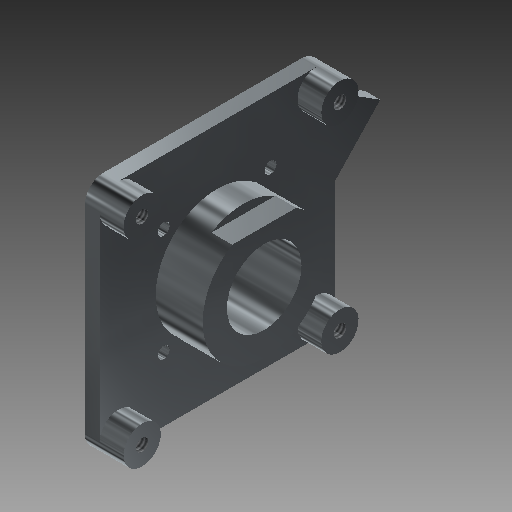
# Autodesk Inventor part: Face Plate
Saved by Autodesk Inventor 2017 (Build 210142000, 142)
## iProperties
Created: 2012-08-06
Part Number: Face Plate
Material: PC/ABS Plastic
Document SubType Name: Modeling
Designer: John
Density: 1.493 g/cm^3
Mass: 11.4166 g
Surface Area: 57.4511 cm^2
Volume: 7.64678 cm^3
Appearance: Zinc
Author: John
Autodesk Inventor part; units mm, degrees
ref_plane "YZ Plane" through (0, 0, 0) normal (1, 0, 0) x (0, 1, 0)
ref_plane "XZ Plane" through (0, 0, 0) normal (0, 1, 0) x (-1, 0, 0)
ref_plane "XY Plane" through (0, 0, 0) normal (0, 0, 1) x (1, 0, 0)
sketch "Sketch1" plane through (0, 0, 0) normal (1, 0, 0) x (0, 1, 0)
  line L0 (0, 0) -> (40.005, 0)
  line L1 (40.005, 0) -> (40.005, 40.005)
  line L2 (40.005, 40.005) -> (0, 40.005)
  line L3 (0, 40.005) -> (0, 0)
  dimension "d0" = 40.005
  dimension "d1" = 40.005
  constraints: 8 end point, 2 parallel, 1 horizontal, 1 perpendicular
  measures "d0" distance of L2.end L1.end
  measures "d1" distance of L0.end L1.end
extrude "Extrusion1" add sketch "Sketch1" along normal blind 2.54
fillet "Fillet1" radius 3.175 4 edges at (1.27, 40.005, 40.005) (1.27, 0, 40.005) (1.27, 0, 0) (1.27, 40.005, 0)
sketch "Sketch2" plane through (2.54, 0, 0) normal (1, 0, 0) x (0, 0, -1)
  arc A0 (0, 36.83) -> (-3.175, 40.005) centre (-3.175, 36.83) ccw projected
  arc A1 (-36.83, 40.005) -> (-40.005, 36.83) centre (-36.83, 36.83) ccw projected
  arc A2 (-40.005, 3.175) -> (-36.83, 0) centre (-36.83, 3.175) ccw projected
  arc A3 (-3.175, 0) -> (0, 3.175) centre (-3.175, 3.175) ccw projected
  circle A4 centre (-36.83, 3.175) radius 3.175
  circle A5 centre (-36.83, 36.83) radius 3.175
  circle A6 centre (-3.175, 36.83) radius 3.175
  circle A7 centre (-3.175, 3.175) radius 3.175
  point P0 (0, 0)
  constraints: 4 coincident, 3 horizontal alignment, 1 centre point, 1 concentric, 6 other
extrude "Extrusion2" add sketch "Sketch2" along normal blind 4.064
sketch "Sketch3" plane through (6.604, 3.175, 36.83) normal (1, 0, 0) x (0, 0, -1)
  circle A0 centre (0, 0) radius 3.175 projected
  circle A1 centre (0, 33.655) radius 3.175 projected
  circle A2 centre (33.655, 33.655) radius 3.175 projected
  circle A3 centre (33.655, 0) radius 3.175 projected
  point P0 (36.83, -3.175)
hole "Hole1" at (6.604, 36.83, 36.83) at (6.604, 36.83, 3.175) at (6.604, 3.175, 3.175) at (6.604, 3.175, 36.83) direction (-1, 0, 0) diameter 2.159 end through all
sketch "Sketch4" plane through (2.54, 0, 0) normal (1, 0, 0) x (0, 0, -1)
  arc A0 (-3.175, 40.005) -> (0, 36.83) centre (-3.175, 36.83) ccw projected
  arc A1 (-36.83, 0) -> (-40.005, 3.175) centre (-36.83, 3.175) ccw projected
  line L0 (-10.9093, 10.9093) -> (-29.0957, 10.9093)
  line L1 (-29.0957, 10.9093) -> (-29.0957, 29.0957)
  line L2 (-29.0957, 29.0957) -> (-10.9093, 29.0957)
  line L3 (-10.9093, 29.0957) -> (-10.9093, 10.9093)
  line L4 (-36.83, 3.175) -> (-3.175, 36.83) construction
  line L5 (-10.9093, 10.9093) -> (-29.0957, 29.0957) construction
  point P0 (0, 0)
  point P1 (-20.0025, 20.0025)
  dimension "d14" = 18.1864
  constraints: 12 end point, 2 midpoint, 2 parallel, 2 perpendicular, 1 horizontal
  measures "d14" distance of L1.end L2.end
hole "Hole2" at (2.54, 10.9093, 29.0957) at (2.54, 29.0957, 29.0957) at (2.54, 10.9093, 10.9093) at (2.54, 29.0957, 10.9093) direction (-1, 0, 0) diameter 2.032 end through all
sketch "Sketch5" plane through (2.54, 0, 0) normal (1, 0, 0) x (0, 0, -1)
  circle A0 centre (-10.9093, 10.9093) radius 1.016 projected
  circle A1 centre (-29.0957, 29.0957) radius 1.016 projected
  line L0 (-29.0957, 29.0957) -> (-10.9093, 10.9093) construction
  circle A2 centre (-20.0025, 20.0025) radius 10.4775
  point P0 (0, 0)
  dimension "d23" = 20.955
  constraints: 2 end point, 1 centre point, 1 midpoint
  measures "d23" diameter of A2
extrude "Extrusion3" add sketch "Sketch5" along normal blind 8.001 contours A2
sketch "Sketch6" plane through (10.541, 20.0025, 20.0025) normal (1, 0, 0) x (0, 0, -1)
  circle A0 centre (0, 0) radius 10.4775 projected
  circle A1 centre (0, 0) radius 6.35
  point P0 (20.0025, -20.0025)
  dimension "d27" = 6.35
  constraints: 1 centre point, 1 coincident
  measures "d27" radius of A1
extrude "Extrusion4" cut sketch "Sketch6" against normal through all contours A1
sketch "Sketch7" plane through (10.541, 20.0025, 20.0025) normal (1, 0, 0) x (0, 0, -1)
  circle A0 centre (0, 0) radius 10.4775 projected
  line L0 (-10.4775, -5.4418) -> (-8.9535, -5.4418)
  line L1 (-8.9535, -5.4418) -> (-8.9535, 5.4418)
  line L2 (-8.9535, 5.4418) -> (-10.4775, 5.4418)
  line L3 (-10.4775, 5.4418) -> (-10.4775, -5.4418)
  point P0 (20.0025, -20.0025)
  dimension "d30" = 19.431
  constraints: 8 end point, 2 parallel, 2 point on circle, 1 horizontal, 1 perpendicular, 1 tangent
extrude "Extrusion5" cut sketch "Sketch7" against normal blind 3.556 contours L1 A0 | A0 L3 L2 | L0 L3 A0 picked at (-9.2326, 1.2437)
sketch "Sketch10" plane through (0, 0, 0) normal (-1, 0, 0) x (0, 0, 1)
  line L0 (3.175, 40.005) -> (36.83, 40.005) projected
  line L1 (21.5392, 40.005) -> (29.7434, 47.752)
  line L2 (29.7434, 47.752) -> (34.6202, 40.005)
  line L3 (36.83, 0) -> (3.175, 0) projected
  line L4 (40.005, 36.83) -> (40.005, 3.175) projected
  point P0 (0, 0)
  dimension "d43" = 5.3848
  dimension "d44" = 10.2616
  dimension "d45" = 18.4658
  dimension "d46" = 47.752
  constraints: 4 end point, 2 point on line
  measures "d43" distance from line of L2.end L4
  measures "d44" distance from line of L4 L1.end
  measures "d45" distance from line of L1.start L4
  measures "d46" distance from line of L3 L1.end
extrude "Extrusion8" add sketch "Sketch10" against normal up to surface (2.54 mm away)
equation "\"d1\" = d0"
body "Solid1"
